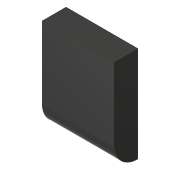
# Autodesk Inventor part: spacer_block
Saved by Autodesk Inventor 2019 (Build 230136000, 136)
## iProperties
Created: 2023-11-21
Part Number: spacer_block
Material: Acetal Resin, Black
Document SubType Name: Modeling
Designer: prich
Mass: 4.37842 g
Surface Area: 15.3226 cm^2
Volume: 3.07257 cm^3
Density: 1.425 g/cm^3
Appearance: Smooth - Black
Author: prich
Autodesk Inventor part; units mm, degrees
ref_plane "YZ Plane" through (0, 0, 0) normal (1, 0, 0) x (0, 1, 0)
ref_plane "XZ Plane" through (0, 0, 0) normal (0, 1, 0) x (-1, 0, 0)
ref_plane "XY Plane" through (0, 0, 0) normal (0, 0, 1) x (1, 0, 0)
sketch "Sketch1" plane through (0, 0, 0) normal (0, 0, 1) x (1, 0, 0)
  line L0 (0, 0) -> (19.05, 0)
  line L1 (19.05, 0) -> (19.05, 25.4)
  line L2 (19.05, 25.4) -> (0, 25.4)
  line L3 (0, 25.4) -> (0, 0)
  dimension "d0" = 19.05
  dimension "d1" = 25.4
  constraints: 8 end point, 2 parallel, 1 horizontal, 1 perpendicular
  measures "d0" distance between parallel lines of L1 L3
  measures "d1" distance between parallel lines of L0 L2
extrude "Extrusion1" add sketch "Sketch1" along normal blind 6.35
fillet "Fillet1" radius 6.35 1 edges at (9.525, 0, 6.35)
body "Solid1"
